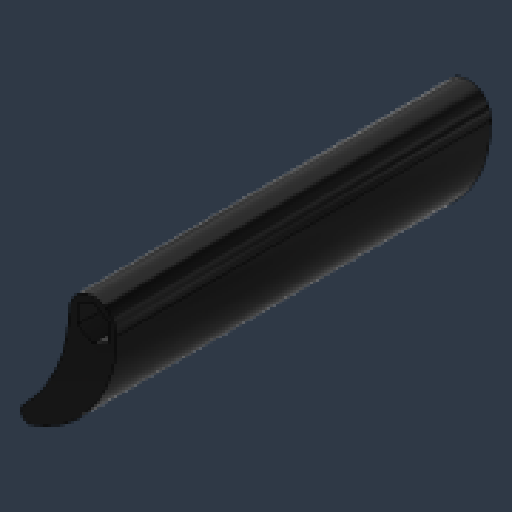
# Autodesk Inventor part: PLATE,TEARDROP,DROPBAR
Saved by Autodesk Inventor 2026 (Build 300175050, 175E)
## iProperties
Created: 2026-04-04
Part Number: PLATE,TEARDROP,DROPBAR
Material: ABS Plastic
Document SubType Name: Modeling
Designer: Jthib
Mass: 135.911 g
Surface Area: 312.777 cm^2
Volume: 128.218 cm^3
Density: 1.06 g/cm^3
Appearance: Smooth - Black
Author: Jthib
Autodesk Inventor part; units mm, degrees
ref_plane "YZ Plane" through (0, 0, 0) normal (1, 0, 0) x (0, 1, 0)
ref_plane "XZ Plane" through (0, 0, 0) normal (0, 1, 0) x (-1, 0, 0)
ref_plane "XY Plane" through (0, 0, 0) normal (0, 0, 1) x (1, 0, 0)
sketch "Sketch1" plane through (0, 0, 0) normal (0, 0, 1) x (1, 0, 0)
  line L0 (-6.35, 3.6662) -> (0, 7.3323)
  line L1 (0, 7.3323) -> (6.35, 3.6662)
  line L2 (6.35, 3.6662) -> (6.35, -3.6662)
  line L3 (6.35, -3.6662) -> (0, -7.3323)
  line L4 (0, -7.3323) -> (-6.35, -3.6662)
  line L5 (-6.35, -3.6662) -> (-6.35, 3.6662)
  arc A0 (9.525, 0.0229) -> (-9.5205, 0.2942) centre (0, 0) ccw
  arc A1 (-38.1, -50.8) -> (-9.5205, 0.2942) centre (-72.9901, 2.2559) ccw
  arc A2 (-38.1, -50.8) -> (9.525, 0.0229) centre (-41.2749, -0.0993) ccw
  dimension "d0" = 12.7
  dimension "d1" = 38.1
  dimension "d2" = 19.05
  dimension "d3" = 50.8
  dimension "d4" = 63.5
  dimension "d5" = 50.8
  constraints: 12 end point, 6 point on circle, 3 centre point, 2 coincident, 2 tangent, 1 vertical, 13 other
  measures "d0" distance between parallel lines of L2 L5
  measures "d1" horizontal distance of point (0, 0) A1.start
  measures "d2" diameter of A0
  measures "d3" vertical distance of point (0, 0) A1.start
  measures "d4" radius of A1
  measures "d5" radius of A2
extrude "Extrusion1" add sketch "Sketch1" along normal mid plane 152.4
fillet "Fillet1" radius 3.175 1 edges at (-38.1, -50.8, 0)
body "Solid1"
